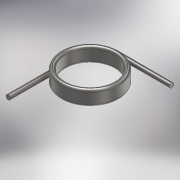
# Autodesk Inventor part: SE03
Saved by Autodesk Inventor 2017 (Build 210142000, 142)
## iProperties
Created: 2019-09-07
Part Number: SE03
Material: Stainless Steel
Document SubType Name: Modeling
Designer: Dell
Density: 8 g/cm^3
Appearance: Semi-Polished
Author: Dell
Autodesk Inventor part; units mm, degrees
ref_plane "YZ Plane" through (0, 0, 0) normal (1, 0, 0) x (0, 1, 0)
ref_plane "XZ Plane" through (0, 0, 0) normal (0, 1, 0) x (-1, 0, 0)
ref_plane "XY Plane" through (0, 0, 0) normal (0, 0, 1) x (1, 0, 0)
sketch "Sketch1" plane through (0, 0, 0) normal (0, 0, 1) x (1, 0, 0)
  circle A0 centre (0, 0) radius 15.494
  circle A1 centre (0, 0) radius 18.415
  dimension "d0" = 30.988
  dimension "d1" = 36.83
  constraints: 2 centre point, 2 coincident
  measures "d0" diameter of A0
  measures "d1" diameter of A1
extrude "Extrusion1" add sketch "Sketch1" along normal blind 9.4933
sketch "Sketch2" plane through (0, 0, 9.4933) normal (0, 0, 1) x (1, 0, 0)
  circle A0 centre (0, 0) radius 15.494 projected
  line L0 (0, 15.494) -> (35, 15.494)
  line L1 (35, 15.494) -> (35, 18.415)
  line L2 (35, 18.415) -> (0, 18.415)
  circle A1 centre (0, 0) radius 18.415 projected
  line L3 (0, 15.494) -> (0, 18.415)
  dimension "d4" = 35
  constraints: 8 end point, 2 horizontal, 2 perpendicular, 1 tangent, 1 vertical, 1 vertical alignment, 1 other
  measures "d4" distance between parallel lines of L1 L3
extrude "Extrusion2" add sketch "Sketch2" against normal blind 2.921 contours L3 A1 L0 | A1 L2 L1 L0 picked at (5.5979, 16.0283)
sketch "Sketch3" plane through (0, 0, 0) normal (0, 0, -1) x (-1, 0, 0)
  line L0 (18.415, 0) -> (18.415, -35)
  line L1 (18.415, -35) -> (15.494, -35)
  line L2 (15.494, -35) -> (15.494, 0)
  circle A0 centre (0, 0) radius 15.494 projected
  line L3 (15.494, 0) -> (18.415, 0)
  circle A1 centre (0, 0) radius 18.415 projected
  point P0 (16.9545, 0)
  dimension "d7" = 35
  constraints: 8 end point, 2 horizontal alignment, 2 perpendicular, 1 midpoint, 1 tangent, 1 vertical, 1 other
  measures "d7" distance between parallel lines of L3 L1
extrude "Extrusion3" add sketch "Sketch3" against normal blind 2.921 contours A1 L2 L3 | L0 L1 L2 A1 picked at (16.0283, -5.5979)
fillet "Fillet1" radius 1.397 16 edges at (17.5, 18.415, 9.4933) (-13.0214, -13.0214, 9.4933) (16.1614, 8.8273, 9.4933) (-18.415, -17.5, 0) (0, 18.415, 0) (5.186, -17.6697, 0) (-15.494, -22.4761, 0) (-15.494, -22.4761, 2.921) (-18.415, -17.5, 2.921) (22.4761, 15.494, 6.5723) (22.4761, 15.494, 9.4933) (17.5, 18.415, 6.5723) (-10.9559, -10.9559, 9.4933) (10.9559, 10.9559, 9.4933) (0, -15.494, 0) (0, 15.494, 0)
body "Solid1"
